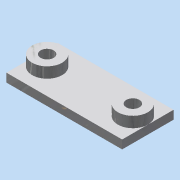
# Autodesk Inventor part: B Oben
Saved by Autodesk Inventor 2015 (Build 190159000, 159)
## iProperties
Created: 2017-11-13
Part Number: B Oben
Material: Generisch
Document SubType Name: Modeling
Designer: Christoph Soppa
Density: 1 g/cm^3
Appearance: Aluminium - poliert
Author: Christoph Soppa
Autodesk Inventor part; units mm, degrees
ref_plane "YZ Plane" through (0, 0, 0) normal (1, 0, 0) x (0, 1, 0)
ref_plane "XZ Plane" through (0, 0, 0) normal (0, 1, 0) x (-1, 0, 0)
ref_plane "XY Plane" through (0, 0, 0) normal (0, 0, 1) x (1, 0, 0)
sketch "Skizze1" plane through (0, 0, 0) normal (0, 0, 1) x (1, 0, 0)
  line L0 (-27, -12) -> (27, -12)
  line L1 (27, -12) -> (27, 12)
  line L2 (27, 12) -> (-27, 12)
  line L3 (-27, 12) -> (-27, -12)
  circle A0 centre (-20, 0) radius 3.05
  circle A1 centre (20, 0) radius 3.05
  point P0 (0, 0)
  dimension "d0" = 54
  dimension "d1" = 24
  dimension "d2" = 12
  dimension "d3" = 27
  dimension "d4" = 6.1
  dimension "d5" = 20
  dimension "d6" = 12
  dimension "d7" = 20
  dimension "d8" = 6.1
  dimension "d9" = 12
  constraints: 8 end point, 2 centre point, 2 parallel, 1 horizontal, 1 perpendicular
  measures "d0" distance of L1.end L2.end
  measures "d1" distance of L0.end L1.end
  measures "d2" distance from line of L2 point (0, 0)
  measures "d3" distance from line of L1 point (0, 0)
  measures "d4" diameter of A0
  measures "d5" distance of point (0, 0) A0.centre
  measures "d6" distance from line of L2 A0.centre
  measures "d7" distance of point (0, 0) A1.centre
  measures "d8" diameter of A1
  measures "d9" distance from line of L2 A1.centre
extrude "Extrusion1" add sketch "Skizze1" along normal blind 4
sketch "Skizze2" plane through (0, 0, 4) normal (0, 0, 1) x (1, 0, 0)
  circle A0 centre (-20, 0) radius 3.05 projected
  circle A1 centre (20, 0) radius 3.05 projected
  circle A2 centre (-20, 0) radius 7
  circle A3 centre (-20, 0) radius 3.05
  circle A4 centre (20, 0) radius 3.05
  circle A5 centre (20, 0) radius 7
  point P0 (0, 0)
  dimension "d3" = 27
  dimension "d12" = 6.1
  dimension "d13" = 14
  dimension "d14" = 6.1
  dimension "d15" = 14
  constraints: 4 centre point, 4 coincident
  measures "d12" diameter of A3
  measures "d13" diameter of A2
  measures "d14" diameter of A4
  measures "d15" diameter of A5
extrude "Extrusion2" add sketch "Skizze2" along normal blind 5
